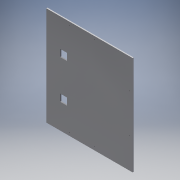
# Autodesk Inventor part: model 2 comp 2 floor part 2
Saved by Autodesk Inventor 2017 (Build 210142000, 142)
## iProperties
Created: 2017-06-12
Part Number: model 2 comp 2 floor part 2
Material: Generic
Document SubType Name: Modeling
Designer: cas7
Density: 1 g/cm^3
Appearance: Default
Author: cas7
Autodesk Inventor part; units mm, degrees
ref_plane "YZ Plane" through (0, 0, 0) normal (1, 0, 0) x (0, 1, 0)
ref_plane "XZ Plane" through (0, 0, 0) normal (0, 1, 0) x (-1, 0, 0)
ref_plane "XY Plane" through (0, 0, 0) normal (0, 0, 1) x (1, 0, 0)
sketch "Sketch1" plane through (0, 0, 0) normal (0, 0, 1) x (1, 0, 0)
  line L0 (0, 0) -> (1219.2, 0)
  line L1 (1219.2, 0) -> (1219.2, 1397)
  line L2 (1219.2, 1397) -> (0, 1397)
  line L3 (0, 1397) -> (0, 0)
  dimension "d0" = 1219.2
  dimension "d1" = 1397
  constraints: 8 end point, 2 parallel, 1 horizontal, 1 perpendicular
  measures "d0" distance of L2.end L1.end
  measures "d1" distance of L1.end L0.end
extrude "Extrusion1" add sketch "Sketch1" along normal blind 15.875
sketch "Sketch8" plane through (0, 0, 15.875) normal (0, 0, 1) x (1, 0, 0)
  line L0 (1219.2, 0) -> (1219.2, 1397) projected
  point P0 (330.9874, 1352.55)
  point P1 (678.6626, 1352.55)
  point P2 (1174.75, 971.55)
  point P3 (1174.75, 425.45)
  point P4 (678.6626, 44.45)
  point P5 (330.9874, 44.45)
  point P6 (330.9874, 1352.55)
  point P7 (678.6626, 1352.55)
  point P8 (1174.75, 971.55)
  point P9 (1174.75, 425.45)
  point P10 (678.6626, 44.45)
  point P11 (330.9874, 44.45)
  constraints: 6 coincident
hole "Hole4" at (330.9874, 1352.55, 15.875) at (678.6626, 1352.55, 15.875) at (1174.75, 971.55, 15.875) at (1174.75, 425.45, 15.875) at (678.6626, 44.45, 15.875) at (330.9874, 44.45, 15.875) direction (0, 0, -1) diameter 10.59 end through all thread size "1/2-13 UNC" class "2B" standard "ANSI Unified Screw Threads"
sketch "Sketch14" plane through (0, 0, 15.875) normal (0, 0, 1) x (1, 0, 0)
  line L0 (1219.2, 0) -> (1219.2, 1397) projected
  line L1 (1219.2, 0) -> (1219.2, 88.9)
  line L2 (1219.2, 88.9) -> (1130.3, 88.9)
  line L3 (1130.3, 88.9) -> (1130.3, 104.775)
  line L4 (1130.3, 104.775) -> (1114.425, 104.775)
  line L5 (1114.425, 104.775) -> (245.225, 104.775)
  line L6 (245.225, 104.775) -> (245.225, 402.275)
  line L7 (295.225, 352.275) -> (195.225, 352.275)
  line L8 (195.225, 352.275) -> (195.225, 452.275)
  line L9 (195.225, 452.275) -> (295.225, 452.275)
  line L10 (295.225, 452.275) -> (295.225, 352.275)
  line L11 (295.225, 352.275) -> (195.225, 452.275) construction
  line L12 (195.225, 352.275) -> (295.225, 452.275) construction
  line L13 (245.225, 104.775) -> (245.225, 948.575)
  line L14 (295.225, 898.575) -> (195.225, 898.575)
  line L15 (195.225, 898.575) -> (195.225, 998.575)
  line L16 (195.225, 998.575) -> (295.225, 998.575)
  line L17 (295.225, 998.575) -> (295.225, 898.575)
  line L18 (295.225, 898.575) -> (195.225, 998.575) construction
  line L19 (195.225, 898.575) -> (295.225, 998.575) construction
  dimension "d80" = 88.9
  dimension "d81" = 88.9
  dimension "d82" = 15.875
  dimension "d83" = 15.875
  dimension "d84" = 869.2
  dimension "d85" = 297.5
  dimension "d86" = 100
  dimension "d87" = 100
  dimension "d88" = 843.8
  dimension "d89" = 100
  dimension "d90" = 100
  constraints: 38 end point, 5 perpendicular, 4 midpoint, 4 parallel, 3 horizontal, 1 point on line, 1 vertical
  measures "d80" distance of L0.start L1.end
  measures "d81" distance of L1.end L2.end
  measures "d82" distance of L2.end L3.end
  measures "d83" distance of L3.end L4.end
  measures "d84" distance of L4.end L5.end
  measures "d85" distance of L5.end L6.end
  measures "d86" distance of L8.end L9.end
  measures "d87" distance of L7.end L8.end
  measures "d88" distance of L5.end L13.end
  measures "d89" distance of L15.end L16.end
  measures "d90" distance of L14.end L15.end
extrude "Extrusion5" cut sketch "Sketch14" against normal blind 15.875
body "Solid1"
